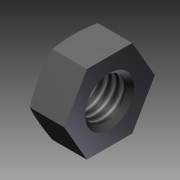
# Autodesk Inventor part: NFJN5nut
Saved by Autodesk Inventor 2011 SP1 (Build 150282100, 282)
## iProperties
Created: 2018-01-07
Part Number: NFJN5nut
Catalog Web Link: www.cadenas.de
Description: NFJN, NFJNS, NFJNFnut-Adjustment Pads - Standard
Vendor: MISUMI
Document SubType Name: Modeling
Designer: psAdmin
Manufacturer: MISUMI
Mass: 0.161835 g
Surface Area: 2.33069 cm^2
Volume: 0.161835 cm^3
Density: 1 g/cm^3
Category: PARTsolutions
Company: MISUMI
Title: NFJN5nut
Author: Cadenas PARTsolutions
Comments: Adjustment Pads - Standard
PSOL_IDENT_0: {$CADENAS_DATA\23d-libs\misumi\metric\42_casters_leveling_pads\nfjn_nut.prj},179 {VTYP=3D},{NB=NFJN5
PSOL_IDENT_1: nut},{LINA=NFJN5nut},{NN=NFJN, NFJNS, NFJNFnut},{DATE=24.04.2017 08:10:58},{GEOMDATE=17.10.2008 07:0
PSOL_IDENT_2: 2:00},{VERSION=},{LINEID=10},{LINESUBID=-1},{WBVAR=TS,MAT}  {NB=NFJN5nut},{LINA=NFJN5nut},{KT=DUMMY}
PSOL_IDENT_3: ,{PN=NFJN5},{TS=1},{TYPE=NFJN},{MAT=1},{M=5},{LL2=4.0},{B=8},{TSA= '1' , 'A Dimension Selectable'  }
PSOL_IDENT_4: ,{MATA= '1', '1018 Steel Equivalent', '2', '304 Stainless Steel' }
NN: NFJN, NFJNS, NFJNFnut
NT: Adjustment Pads - Standard
NB: NFJN5nut
NBSYN: $PN.nut
LINA: NFJN5nut
PN: NFJN5
TS: A Dimension Selectable
MAT: 1018 Steel Equivalent
M: 5
LL2: 4.0
B: 8
SUPPLIER: MISUMI
ARTICLENO: NFJN5nut
BOMINFO: NFJN5nut
CREATOR: CADENAS GmbH
Autodesk Inventor part; units mm, degrees
sketch "Sketch_1" plane through (0, 0, 0) normal (0, 0, 1) x (1, 0, 0)
  line L0 (4, 0) -> (0, 0)
  line L1 (0, 2.5) -> (0.433, 2.067)
  line L2 (0.433, 2.067) -> (3.567, 2.067)
  line L3 (3.567, 2.067) -> (4, 2.5)
  line L4 (4, 2.5) -> (4, 5)
  line L5 (4, 5) -> (0.6154, 5)
  line L6 (0.6154, 5) -> (0, 3.3333)
  line L7 (0, 3.3333) -> (0, 2.5)
  constraints: 16 end point
revolve "Revolution1" add sketch "Sketch_1" angle 360 about axis through (4, 0, 0) along (1, 0, 0)
thread "Thread1" size "M5x0.8" class "6H" standard "ISO Metric profile" full length
sketch "Sketch_2" plane through (0, 0, 0) normal (1, 0, 0) x (0, 1, 0)
  line L0 (-4.6188, 8) -> (-9.2376, 0)
  line L1 (-9.2376, 0) -> (-4.6188, -8)
  line L2 (-4.6188, -8) -> (4.6188, -8)
  line L3 (4.6188, -8) -> (9.2376, 0)
  line L4 (9.2376, 0) -> (4.6188, 8)
  line L5 (4.6188, 8) -> (-4.6188, 8)
  line L6 (-2.3094, 4) -> (-4.6188, 0)
  line L7 (-4.6188, 0) -> (-2.3094, -4)
  line L8 (-2.3094, -4) -> (2.3094, -4)
  line L9 (2.3094, -4) -> (4.6188, 0)
  line L10 (4.6188, 0) -> (2.3094, 4)
  line L11 (2.3094, 4) -> (-2.3094, 4)
  constraints: 24 end point
extrude "Extrusion1" cut sketch "Sketch_2" along normal blind 4
ref_plane "nut_to_pad_XY" through (0, 0, 0) normal (1, 0, 0) x (0, 0, -1)
ref_plane "nut_to_pad_YZ" through (0, 0, 0) normal (0, 0, -1) x (0, 1, 0)
ref_plane "nut_to_pad_ZX" through (0, 0, 0) normal (0, 1, 0) x (1, 0, 0)
body "Solid1"
